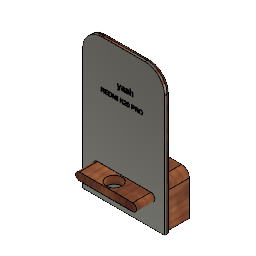
yyyyy (Autodesk Fusion 360 design; units mm, degrees)
Autodesk Fusion 360 part; units mm, degrees
sketch "Sketch1" plane through (0, 0, 0) normal (0, 0, 1) x (1, 0, 0) in component "back"
  line L0 (0, 40) -> (25, 40)
  line L1 (25, 40) -> (25, 35)
  line L2 (25, 35) -> (0, 35)
  line L3 (0, 35) -> (0, 40)
  constraint horizontal L0
  constraint vertical L1
  constraint horizontal L2
  constraint vertical L3
extrude "Extrude1" add sketch "Sketch1" along normal blind 180 makes body 1 in component "back"
extrude "Extrude2" add 1 faces at (25, 38.3333, 60) along direction (1, 0, 0) blind 80 on bodies 1 bodies 1 in component "back"
sketch "Sketch1 (2)" plane through (0, 0, 0) normal (0, 0, 1) x (1, 0, 0) in component "cube"
  line L0 (50, 70) -> (70, 70)
  line L1 (70, 70) -> (70, 50)
  line L2 (70, 50) -> (50, 50)
  line L3 (50, 50) -> (50, 70)
  constraint horizontal L0
  constraint vertical L1
  constraint horizontal L2
  constraint vertical L3
extrude "Extrude1'" add sketch "Sketch1 (2)" along normal blind 35 separate body makes body 2 in component "cube"
extrude "Extrude2'" add 1 faces at (50, 56.6667, 23.3333) along direction (-1, 0, 0) blind 45 on bodies 2 bodies 2 in component "cube"
extrude "Extrude3" add 1 faces at (70, 63.3333, 23.3333) along direction (1, 0, 0) blind 35 on bodies 2 bodies 2 in component "cube"
move_body "Move1" bodies 2 to x (1, 0, 0) y (0, 1, 0) z (0, 0, 1) at (0, -10, 0) in component "cube"
extrude "Extrude4" add 1 faces at (38.3333, 60, 11.6667) along direction (0, 1, 0) blind 10 on bodies 2 bodies 2 in component "cube"
extrude "Extrude5" add 1 faces at (38.3333, 60, 35) along direction (0, 0, 1) blind 20 on bodies 2 bodies 2 in component "cube"
fillet "Fillet1" radius 25 1 edges at (105, 37.5, 180) on bodies 1 in component "back"
fillet "Fillet2" radius 25 1 edges at (0, 37.5, 180) on bodies 1 in component "back"
sketch "Sketch1 (3)" plane through (0, 0, 0) normal (0, 0, 1) x (1, 0, 0)
  line L0 (-153.9554, 34.6493) -> (-75.6667, 34.6493)
  line L1 (-75.6667, 34.6493) -> (-75.6667, 11.4249)
  line L2 (-75.6667, 11.4249) -> (-153.9554, 11.4249)
  line L3 (-153.9554, 11.4249) -> (-153.9554, 34.6493)
  constraint horizontal L0
  constraint vertical L1
  constraint horizontal L2
  constraint vertical L3
extrude "Extrude1''" add sketch "Sketch1 (3)" along normal blind 10 separate body makes body 3
move_body "Move1'" bodies 3 to x (1, 0, 0) y (0, 1, 0) z (0, 0, 1) at (168.4842, 0, 29.5709)
hole "Hole1" at (52.551, 22.9766, 39.5709) direction (0, 0, -1) diameter 20 depth 30 tip angle 118 bodies 3
sketch "Sketch2" plane through (0, 0, 55) normal (0, 0, 1) x (-1, 0, 0)
  line L0 (-5, -40) -> (-105, -40)
  line L1 (-105, -40) -> (-105, -70)
  line L2 (-105, -70) -> (-5, -70)
  line L3 (-5, -70) -> (-5, -40)
  line L4 (40, -110) -> (-23.3941, -110)
  line L5 (-23.3941, -110) -> (-23.3941, -80.2857)
  line L6 (-23.3941, -80.2857) -> (40, -80.2857)
  line L7 (40, -80.2857) -> (40, -110)
  constraint horizontal L4
  constraint vertical L5
  constraint horizontal L6
  constraint vertical L7
shell "Shell1" thickness 5 removed faces 1 at (38.3333, 70, 36.6667) on bodies 2 in component "cube"
move_body "Move2" bodies 2 to x (1, 0, 0) y (0, 1, 0) z (0, 0, 1) at (-3, 0, 0) in component "cube"
fillet "Fillet1'" radius 5 1 edges at (92.8175, 23.0371, 39.5709) on bodies 3
fillet "Fillet2'" radius 5 1 edges at (14.5288, 23.0371, 39.5709) on bodies 3
fillet "Fillet1''" radius 10 1 edges at (2, 55, 55) on bodies 2 in component "cube"
fillet "Fillet2''" radius 10 1 edges at (102, 55, 55) on bodies 2 in component "cube"
fillet "Fillet3" radius 5 1 edges at (92.8175, 23.0371, 29.5709) on bodies 3
fillet "Fillet4" radius 5 1 edges at (14.5288, 23.0371, 29.5709) on bodies 3
sketch "Sketch1 (4)" plane through (0, 35, 0) normal (0, -1, 0) x (1, 0, 0) in component "name"
  arc A0 (25, 180) -> (0, 155) centre (25, 155) ccw
  line L0 (0, 155) -> (0, 0)
  line L1 (0, 0) -> (105, 0)
  line L2 (105, 0) -> (105, 155)
  arc A1 (105, 155) -> (80, 180) centre (80, 155) ccw
  line L3 (80, 180) -> (25, 180)
  line L4 (44.3127, 130.9182) -> (64.596, 130.9182) construction
  line L5 (64.596, 130.9182) -> (64.596, 140.9182) construction
  line L6 (64.596, 140.9182) -> (44.3127, 140.9182) construction
  line L7 (44.3127, 140.9182) -> (44.3127, 130.9182) construction
  text T0 "yash" font "Arial" height 10 align ink ink in box 0 x 0 at (44.3127, 130.9182) x (1, 0) y (0, 1) spacing 1 height is em
  constraint perpendicular L4 L5
  constraint parallel L4 L6
  constraint parallel L5 L7
sketch "Sketch2 (2)" plane through (0, 0, 0) normal (0, 1, 0) x (1, 0, 0) in component "name"
  line L0 (31.1731, -116.0159, 40) -> (73.9514, -116.0159, 40) construction
  line L1 (73.9514, -116.0159, 40) -> (73.9514, -126.0159, 40) construction
  line L2 (73.9514, -126.0159, 40) -> (31.1731, -126.0159, 40) construction
  line L3 (31.1731, -126.0159, 40) -> (31.1731, -116.0159, 40) construction
extrude "Extrude3'" cut sketch "Sketch1 (4)" against normal blind 3 text T0 bodies 1 in component "back"
extrude "Extrude1'''" add 1 faces at (50.1868, 35, 43.648) along direction (0, 1, 0) blind 3 separate body on bodies 1 makes body 4 in component "name"
sketch "Sketch1 (5)" plane through (0, 35, 0) normal (0, -1, 0) x (1, 0, 0) in component "Component"
  arc A0 (25, 180) -> (0, 155) centre (25, 155) ccw
  line L0 (0, 155) -> (0, 0)
  line L1 (0, 0) -> (105, 0)
  line L2 (105, 0) -> (105, 155)
  arc A1 (105, 155) -> (80, 180) centre (80, 155) ccw
  line L3 (80, 180) -> (25, 180)
  spline S0 degree 3 poles (46.0708, 131.1308) (45.9625, 131.0717) (45.7375, 130.9489) (45.4812, 130.9352) (45.3481, 130.9282) knots 0 0 0 0 0.036516 0.075906 0.075906 0.075906 0.075906
  spline S1 degree 3 poles (45.3481, 130.9282) (45.258, 130.9337) (45.0648, 130.9456) (44.8802, 131.0043) (44.7817, 131.0356) knots 0 0 0 0 0.026989 0.057845 0.057845 0.057845 0.057845
  line L4 (44.7817, 131.0356) -> (44.6841, 131.8608)
  spline S2 degree 3 poles (44.6841, 131.8608) (44.7735, 131.838) (44.9388, 131.796) (45.1089, 131.7869) (45.187, 131.7827) knots 0 0 0 0 0.027607 0.051004 0.051004 0.051004 0.051004
  spline S3 degree 3 poles (45.187, 131.7827) (45.2762, 131.7849) (45.4388, 131.7889) (45.5883, 131.8519) (45.6558, 131.8803) knots 0 0 0 0 0.02648 0.048256 0.048256 0.048256 0.048256
  spline S4 degree 3 poles (45.6558, 131.8803) (45.7119, 131.9164) (45.8252, 131.9893) (45.904, 132.0986) (45.9438, 132.1537) knots 0 0 0 0 0.019825 0.040035 0.040035 0.040035 0.040035
  spline S5 degree 3 poles (45.9438, 132.1537) (45.9812, 132.2298) (46.0854, 132.4416) (46.1628, 132.6649) (46.2124, 132.808) knots 0 0 0 0 0.025391 0.070782 0.070782 0.070782 0.070782
  spline S6 degree 3 poles (46.2124, 132.808) (46.2229, 132.8382) (46.2478, 132.9102) (46.2748, 132.9815) (46.2905, 133.0229) knots 0 0 0 0 0.009575 0.022862 0.022862 0.022862 0.022862
  line L5 (46.2905, 133.0229) -> (44.3227, 138.2182)
  line L6 (44.3227, 138.2182) -> (45.27, 138.2182)
  line L7 (45.27, 138.2182) -> (46.3491, 135.2153)
  spline S7 degree 3 poles (46.3491, 135.2153) (46.4177, 135.0207) (46.5573, 134.6248) (46.6685, 134.2199) (46.7251, 134.0141) knots 0 0 0 0 0.06188 0.125899 0.125899 0.125899 0.125899
  spline S8 degree 3 poles (46.7251, 134.0141) (46.7778, 134.2143) (46.8829, 134.6129) (47.0188, 135.002) (47.0864, 135.1957) knots 0 0 0 0 0.062076 0.123607 0.123607 0.123607 0.123607
  line L8 (47.0864, 135.1957) -> (48.1948, 138.2182)
  line L9 (48.1948, 138.2182) -> (49.0737, 138.2182)
  line L10 (49.0737, 138.2182) -> (47.1011, 132.9448)
  spline S9 degree 3 poles (47.1011, 132.9448) (47.0115, 132.7024) (46.8639, 132.303) (46.6802, 131.919) (46.6079, 131.768) knots 0 0 0 0 0.077459 0.12765 0.12765 0.12765 0.12765
  spline S10 degree 3 poles (46.6079, 131.768) (46.5315, 131.6361) (46.39, 131.3914) (46.1715, 131.213) (46.0708, 131.1308) knots 0 0 0 0 0.045283 0.08395 0.08395 0.08395 0.08395
  line L11 (61.2612, 135.8696) -> (61.2612, 133.0327)
  line L12 (61.2612, 133.0327) -> (60.3823, 133.0327)
  line L13 (60.3823, 133.0327) -> (60.3823, 140.1909)
  line L14 (60.3823, 140.1909) -> (61.2612, 140.1909)
  line L15 (61.2612, 140.1909) -> (61.2612, 137.6225)
  spline S11 degree 3 poles (61.2612, 137.6225) (61.4795, 137.8304) (61.9156, 138.2457) (62.5148, 138.3055) (62.814, 138.3354) knots 0 0 0 0 0.08775 0.175277 0.175277 0.175277 0.175277
  spline S12 degree 3 poles (62.814, 138.3354) (62.996, 138.3278) (63.344, 138.3134) (63.6629, 138.1745) (63.8149, 138.1083) knots 0 0 0 0 0.054131 0.103431 0.103431 0.103431 0.103431
  spline S13 degree 3 poles (63.8149, 138.1083) (63.9457, 138.0271) (64.2009, 137.8686) (64.3501, 137.608) (64.4228, 137.4809) knots 0 0 0 0 0.045374 0.088594 0.088594 0.088594 0.088594
  spline S14 degree 3 poles (64.4228, 137.4809) (64.476, 137.3186) (64.5993, 136.9419) (64.6036, 136.5448) (64.606, 136.3188) knots 0 0 0 0 0.050958 0.118252 0.118252 0.118252 0.118252
  line L16 (64.606, 136.3188) -> (64.606, 133.0327)
  line L17 (64.606, 133.0327) -> (63.727, 133.0327)
  line L18 (63.727, 133.0327) -> (63.727, 136.3188)
  spline S15 degree 3 poles (63.727, 136.3188) (63.7225, 136.5148) (63.7144, 136.8629) (63.5244, 137.152) (63.4414, 137.2783) knots 0 0 0 0 0.057392 0.10189 0.10189 0.10189 0.10189
  spline S16 degree 3 poles (63.4414, 137.2783) (63.3313, 137.3657) (63.0956, 137.5529) (62.794, 137.5696) (62.6333, 137.5785) knots 0 0 0 0 0.041188 0.088118 0.088118 0.088118 0.088118
  spline S17 degree 3 poles (62.6333, 137.5785) (62.5047, 137.5699) (62.2459, 137.5525) (62.0147, 137.435) (61.8984, 137.3759) knots 0 0 0 0 0.03824 0.076933 0.076933 0.076933 0.076933
  spline S18 degree 3 poles (61.8984, 137.3759) (61.7923, 137.3033) (61.5835, 137.1604) (61.4657, 136.9367) (61.4077, 136.8266) knots 0 0 0 0 0.037929 0.074658 0.074658 0.074658 0.074658
  spline S19 degree 3 poles (61.4077, 136.8266) (61.3651, 136.69) (61.2682, 136.379) (61.2637, 136.0526) (61.2612, 135.8696) knots 0 0 0 0 0.042697 0.097264 0.097264 0.097264 0.097264
  spline S20 degree 3 poles (57.2476, 132.9155) (56.943, 132.9241) (56.3931, 132.9396) (55.9187, 133.2133) (55.707, 133.3354) knots 0 0 0 0 0.089667 0.161897 0.161897 0.161897 0.161897
  spline S21 degree 3 poles (55.707, 133.3354) (55.5452, 133.4996) (55.2013, 133.8485) (55.0898, 134.3271) (55.0308, 134.5805) knots 0 0 0 0 0.067824 0.14416 0.14416 0.14416 0.14416
  line L19 (55.0308, 134.5805) -> (55.8999, 134.7172)
  spline S22 degree 3 poles (55.8999, 134.7172) (55.932, 134.556) (55.9929, 134.25) (56.2065, 134.0236) (56.3076, 133.9164) knots 0 0 0 0 0.048178 0.091492 0.091492 0.091492 0.091492
  spline S23 degree 3 poles (56.3076, 133.9164) (56.4377, 133.8354) (56.7227, 133.6579) (57.0595, 133.6451) (57.2427, 133.6381) knots 0 0 0 0 0.045208 0.099065 0.099065 0.099065 0.099065
  spline S24 degree 3 poles (57.2427, 133.6381) (57.4233, 133.6423) (57.7451, 133.6497) (58.0204, 133.8131) (58.1411, 133.8847) knots 0 0 0 0 0.053093 0.094556 0.094556 0.094556 0.094556
  spline S25 degree 3 poles (58.1411, 133.8847) (58.2265, 133.968) (58.3906, 134.128) (58.42, 134.3547) (58.4341, 134.4633) knots 0 0 0 0 0.034652 0.06657 0.06657 0.06657 0.06657
  spline S26 degree 3 poles (58.4341, 134.4633) (58.4228, 134.5576) (58.3999, 134.7486) (58.2508, 134.8704) (58.1753, 134.9321) knots 0 0 0 0 0.027386 0.055446 0.055446 0.055446 0.055446
  spline S27 degree 3 poles (58.1753, 134.9321) (58.0712, 134.9788) (57.7823, 135.1085) (57.474, 135.1826) (57.2768, 135.2299) knots 0 0 0 0 0.034189 0.094822 0.094822 0.094822 0.094822
  spline S28 degree 3 poles (57.2768, 135.2299) (57.0018, 135.2988) (56.5463, 135.4129) (56.1095, 135.5844) (55.9365, 135.6523) knots 0 0 0 0 0.084955 0.140654 0.140654 0.140654 0.140654
  spline S29 degree 3 poles (55.9365, 135.6523) (55.8206, 135.7157) (55.5955, 135.8388) (55.4437, 136.0453) (55.3701, 136.1454) knots 0 0 0 0 0.039108 0.075916 0.075916 0.075916 0.075916
  spline S30 degree 3 poles (55.3701, 136.1454) (55.3139, 136.2537) (55.2004, 136.4719) (55.185, 136.7175) (55.1772, 136.8412) knots 0 0 0 0 0.036161 0.072917 0.072917 0.072917 0.072917
  spline S31 degree 3 poles (55.1772, 136.8412) (55.1836, 136.9542) (55.1963, 137.1783) (55.2896, 137.3822) (55.3359, 137.4833) knots 0 0 0 0 0.033621 0.066662 0.066662 0.066662 0.066662
  spline S32 degree 3 poles (55.3359, 137.4833) (55.3936, 137.5777) (55.5091, 137.7664) (55.6817, 137.9048) (55.7681, 137.9741) knots 0 0 0 0 0.032897 0.065829 0.065829 0.065829 0.065829
  spline S33 degree 3 poles (55.7681, 137.9741) (55.8473, 138.0239) (56.0222, 138.1339) (56.2193, 138.1963) (56.3271, 138.2304) knots 0 0 0 0 0.027973 0.061727 0.061727 0.061727 0.061727
  spline S34 degree 3 poles (56.3271, 138.2304) (56.4488, 138.261) (56.698, 138.3237) (56.9549, 138.3314) (57.0864, 138.3354) knots 0 0 0 0 0.037518 0.076851 0.076851 0.076851 0.076851
  spline S35 degree 3 poles (57.0864, 138.3354) (57.279, 138.3298) (57.6444, 138.3192) (57.9932, 138.2108) (58.1582, 138.1596) knots 0 0 0 0 0.05748 0.109059 0.109059 0.109059 0.109059
  spline S36 degree 3 poles (58.1582, 138.1596) (58.2986, 138.1001) (58.56, 137.9894) (58.751, 137.7803) (58.8393, 137.6835) knots 0 0 0 0 0.045124 0.083974 0.083974 0.083974 0.083974
  spline S37 degree 3 poles (58.8393, 137.6835) (58.9078, 137.5691) (59.0567, 137.32) (59.1121, 137.0346) (59.1421, 136.8803) knots 0 0 0 0 0.039698 0.086419 0.086419 0.086419 0.086419
  line L20 (59.1421, 136.8803) -> (58.2827, 136.7631)
  spline S38 degree 3 poles (58.2827, 136.7631) (58.2555, 136.8879) (58.2029, 137.1296) (58.028, 137.3039) (57.9434, 137.3881) knots 0 0 0 0 0.037427 0.072477 0.072477 0.072477 0.072477
  spline S39 degree 3 poles (57.9434, 137.3881) (57.8332, 137.4535) (57.5897, 137.598) (57.3055, 137.6075) (57.1499, 137.6127) knots 0 0 0 0 0.037832 0.083649 0.083649 0.083649 0.083649
  spline S40 degree 3 poles (57.1499, 137.6127) (56.973, 137.6113) (56.6683, 137.6088) (56.3987, 137.4706) (56.2856, 137.4125) knots 0 0 0 0 0.052121 0.089788 0.089788 0.089788 0.089788
  spline S41 degree 3 poles (56.2856, 137.4125) (56.2102, 137.3458) (56.0676, 137.2197) (56.0399, 137.0321) (56.0268, 136.9438) knots 0 0 0 0 0.029135 0.0551 0.0551 0.0551 0.0551
  spline S42 degree 3 poles (56.0268, 136.9438) (56.0314, 136.8881) (56.0406, 136.7763) (56.1029, 136.683) (56.1343, 136.6362) knots 0 0 0 0 0.016456 0.033067 0.033067 0.033067 0.033067
  spline S43 degree 3 poles (56.1343, 136.6362) (56.178, 136.5899) (56.2738, 136.4886) (56.4017, 136.4324) (56.4712, 136.4018) knots 0 0 0 0 0.018913 0.04141 0.04141 0.04141 0.04141
  spline S44 degree 3 poles (56.4712, 136.4018) (56.5577, 136.3745) (56.8147, 136.2935) (57.075, 136.2236) (57.2476, 136.1772) knots 0 0 0 0 0.027221 0.080828 0.080828 0.080828 0.080828
  spline S45 degree 3 poles (57.2476, 136.1772) (57.513, 136.1067) (57.9529, 135.9899) (58.3796, 135.832) (58.5488, 135.7695) knots 0 0 0 0 0.082338 0.13643 0.13643 0.13643 0.13643
  spline S46 degree 3 poles (58.5488, 135.7695) (58.6643, 135.7118) (58.89, 135.5989) (59.0495, 135.4035) (59.1274, 135.308) knots 0 0 0 0 0.038228 0.07476 0.07476 0.07476 0.07476
  spline S47 degree 3 poles (59.1274, 135.308) (59.1886, 135.1974) (59.3179, 134.9638) (59.3307, 134.6967) (59.3374, 134.5561) knots 0 0 0 0 0.037411 0.079003 0.079003 0.079003 0.079003
  spline S48 degree 3 poles (59.3374, 134.5561) (59.3261, 134.4108) (59.3031, 134.1157) (59.1558, 133.8588) (59.081, 133.7285) knots 0 0 0 0 0.043142 0.087613 0.087613 0.087613 0.087613
  spline S49 degree 3 poles (59.081, 133.7285) (58.9836, 133.6053) (58.7819, 133.3504) (58.4914, 133.2037) (58.3413, 133.1279) knots 0 0 0 0 0.046534 0.096306 0.096306 0.096306 0.096306
  spline S50 degree 3 poles (58.3413, 133.1279) (58.1713, 133.0659) (57.8182, 132.9373) (57.4425, 132.9229) (57.2476, 132.9155) knots 0 0 0 0 0.053921 0.112025 0.112025 0.112025 0.112025
  line L21 (54.2983, 133.0327) -> (53.3804, 133.0327)
  spline S51 degree 3 poles (53.3804, 133.0327) (53.3386, 133.1303) (53.2509, 133.3354) (53.2205, 133.5565) (53.2046, 133.6723) knots 0 0 0 0 0.031718 0.066602 0.066602 0.066602 0.066602
  spline S52 degree 3 poles (53.2046, 133.6723) (53.0496, 133.5466) (52.7604, 133.312) (52.4218, 133.1579) (52.2646, 133.0864) knots 0 0 0 0 0.059572 0.111161 0.111161 0.111161 0.111161
  spline S53 degree 3 poles (52.2646, 133.0864) (52.1099, 133.0365) (51.7947, 132.935) (51.4638, 132.9221) (51.2954, 132.9155) knots 0 0 0 0 0.048537 0.098829 0.098829 0.098829 0.098829
  spline S54 degree 3 poles (51.2954, 132.9155) (51.0353, 132.9259) (50.5572, 132.945) (50.1621, 133.2114) (49.9819, 133.3329) knots 0 0 0 0 0.076279 0.140251 0.140251 0.140251 0.140251
  spline S55 degree 3 poles (49.9819, 133.3329) (49.8481, 133.4831) (49.5768, 133.7875) (49.5411, 134.194) (49.5229, 134.3998) knots 0 0 0 0 0.0587 0.118946 0.118946 0.118946 0.118946
  spline S56 degree 3 poles (49.5229, 134.3998) (49.5297, 134.5232) (49.5431, 134.7663) (49.6457, 134.987) (49.6963, 135.0956) knots 0 0 0 0 0.036695 0.072295 0.072295 0.072295 0.072295
  spline S57 degree 3 poles (49.6963, 135.0956) (49.7578, 135.1949) (49.879, 135.3906) (50.0609, 135.5316) (50.1504, 135.601) knots 0 0 0 0 0.034732 0.06843 0.06843 0.06843 0.06843
  spline S58 degree 3 poles (50.1504, 135.601) (50.248, 135.6609) (50.4468, 135.783) (50.6694, 135.8533) (50.7827, 135.8891) knots 0 0 0 0 0.034212 0.069718 0.069718 0.069718 0.069718
  spline S59 degree 3 poles (50.7827, 135.8891) (50.8907, 135.9129) (51.1488, 135.9698) (51.4113, 136.0021) (51.564, 136.0209) knots 0 0 0 0 0.033158 0.079268 0.079268 0.079268 0.079268
  spline S60 degree 3 poles (51.564, 136.0209) (51.8738, 136.0584) (52.4037, 136.1226) (52.9178, 136.2647) (53.1313, 136.3237) knots 0 0 0 0 0.093449 0.159827 0.159827 0.159827 0.159827
  spline S61 degree 3 poles (53.1313, 136.3237) (53.1327, 136.3729) (53.1349, 136.4494) (53.1359, 136.5259) (53.1362, 136.5532) knots 0 0 0 0 0.014775 0.022955 0.022955 0.022955 0.022955
  spline S62 degree 3 poles (53.1362, 136.5532) (53.1327, 136.712) (53.1265, 136.992) (52.9595, 137.2139) (52.8872, 137.31) knots 0 0 0 0 0.046198 0.081458 0.081458 0.081458 0.081458
  spline S63 degree 3 poles (52.8872, 137.31) (52.7515, 137.3966) (52.448, 137.5904) (52.0862, 137.6016) (51.8862, 137.6078) knots 0 0 0 0 0.047457 0.106158 0.106158 0.106158 0.106158
  spline S64 degree 3 poles (51.8862, 137.6078) (51.7026, 137.605) (51.3799, 137.6) (51.094, 137.4536) (50.9707, 137.3906) knots 0 0 0 0 0.054167 0.095201 0.095201 0.095201 0.095201
  spline S65 degree 3 poles (50.9707, 137.3906) (50.8766, 137.2953) (50.6632, 137.0792) (50.5801, 136.7856) (50.5337, 136.6215) knots 0 0 0 0 0.039569 0.089726 0.089726 0.089726 0.089726
  line L22 (50.5337, 136.6215) -> (49.6743, 136.7387)
  spline S66 degree 3 poles (49.6743, 136.7387) (49.7162, 136.9092) (49.7947, 137.2284) (49.9757, 137.5023) (50.0601, 137.6298) knots 0 0 0 0 0.05222 0.097745 0.097745 0.097745 0.097745
  spline S67 degree 3 poles (50.0601, 137.6298) (50.164, 137.738) (50.3847, 137.9677) (50.6801, 138.0884) (50.8364, 138.1523) knots 0 0 0 0 0.044497 0.094504 0.094504 0.094504 0.094504
  spline S68 degree 3 poles (50.8364, 138.1523) (51.0179, 138.2056) (51.4018, 138.3185) (51.8021, 138.3296) (52.0132, 138.3354) knots 0 0 0 0 0.056504 0.119536 0.119536 0.119536 0.119536
  spline S69 degree 3 poles (52.0132, 138.3354) (52.2153, 138.332) (52.582, 138.3258) (52.9342, 138.2246) (53.0923, 138.1791) knots 0 0 0 0 0.060307 0.109454 0.109454 0.109454 0.109454
  spline S70 degree 3 poles (53.0923, 138.1791) (53.2175, 138.1282) (53.4461, 138.0352) (53.6228, 137.8636) (53.7026, 137.7861) knots 0 0 0 0 0.040099 0.0732 0.0732 0.0732 0.0732
  spline S71 degree 3 poles (53.7026, 137.7861) (53.7634, 137.6993) (53.8911, 137.5169) (53.9469, 137.3011) (53.9761, 137.1879) knots 0 0 0 0 0.031521 0.066244 0.066244 0.066244 0.066244
  spline S72 degree 3 poles (53.9761, 137.1879) (53.9887, 137.083) (54.0212, 136.814) (54.0205, 136.5428) (54.02, 136.3774) knots 0 0 0 0 0.031666 0.081239 0.081239 0.081239 0.081239
  line L23 (54.02, 136.3774) -> (54.02, 135.2055)
  spline S73 degree 3 poles (54.02, 135.2055) (54.018, 134.8717) (54.0149, 134.354) (54.0601, 133.8384) (54.0762, 133.6552) knots 0 0 0 0 0.100046 0.1552 0.1552 0.1552 0.1552
  spline S74 degree 3 poles (54.0762, 133.6552) (54.0997, 133.5477) (54.1472, 133.3307) (54.2477, 133.1326) (54.2983, 133.0327) knots 0 0 0 0 0.03288 0.06634 0.06634 0.06634 0.06634
  line L24 (23.8329, 118.8443) -> (77.037, 118.8443) construction
  line L25 (77.037, 118.8443) -> (77.037, 125.8443) construction
  line L26 (77.037, 125.8443) -> (23.8329, 125.8443) construction
  line L27 (23.8329, 125.8443) -> (23.8329, 118.8443) construction
  text T0 "REDMI K20 PRO" font "Arial" height 7 align ink ink in box 0 x 0 at (23.8329, 118.8443) x (1, 0) y (0, 1) spacing 1 height is em
  constraint perpendicular L24 L25
  constraint parallel L24 L26
  constraint parallel L25 L27
extrude "Extrude1''''" add sketch "Sketch1 (5)" against normal blind 2 separate body text T0 makes body 5 at (28.9015, 35.6667, 120.62) makes body 6 at (43.1601, 35, 122.018) makes body 7 at (72.5078, 35, 121.7376) makes body 8 at (54.8815, 35.6667, 118.9498) makes body 9 at (62.7326, 35.6667, 120.62) makes body 10 at (67.4118, 35.6667, 120.62) makes body 11 at (57.0804, 35, 120.982) makes body 12 at (48.3053, 35.6667, 120.62) makes body 13 at (44.5558, 35.6667, 120.62) makes body 14 at (33.5568, 35.6667, 120.62) makes body 15 at (23.8429, 35.6667, 120.62) in component "Component"
component "back" placed x (1, 0, 0) y (0, 1, 0) z (0, 0, 1) at (0, 0, 0)
component "cube" placed x (1, 0, 0) y (0, 1, 0) z (0, 0, 1) at (0, 0, 0)
component "name" placed x (1, 0, 0) y (0, 1, 0) z (0, 0, 1) at (0, 0, 0)
component "Component" placed x (1, 0, 0) y (0, 1, 0) z (0, 0, 1) at (0, 0, 0)
equation "le = 180 mm"
equation "widt = 80 mm"
equation "th = 6.25 mm"
equation "d5 = le"
equation "d7 = widt"
equation "slit = 60 mm"
